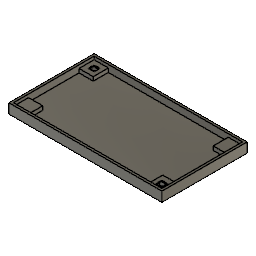
PCB_PDP_TD01_GP09 v1 (Autodesk Fusion 360 archive; units mm, degrees)
design "dessous"
Autodesk Fusion 360 part; units mm, degrees
sketch "Sketch1" plane through (0, 0, 0) normal (0, 0, 1) x (1, 0, 0)
  line L0 (-39.5, 22) -> (39.5, 22)
  line L1 (39.5, 22) -> (39.5, -22)
  line L2 (39.5, -22) -> (-39.5, -22)
  line L3 (-39.5, -22) -> (-39.5, 22)
  dimension "d1" = 79
  dimension "d2" = 44
  dimension "d3" = 39.5
  dimension "d4" = 22
  constraint horizontal L0
  constraint vertical L1
  constraint horizontal L2
  constraint vertical L3
  measures "d1" distance of L0.start L0.end
  measures "d2" distance of L0.start L2.end
  measures "d3" distance of origin L3
  measures "d4" distance of origin L0
extrude "Extrude1" add sketch "Sketch1" along normal blind 4.8
sketch "Sketch2" plane through (0, 0, 4.8) normal (0, 0, 1) x (-1, 0, 0)
  line L0 (39.5, 22) -> (-39.5, 22)
  line L1 (-39.5, 22) -> (-39.5, -22)
  line L2 (-39.5, -22) -> (39.5, -22)
  line L3 (39.5, -22) -> (39.5, 22)
  line L4 (38.3, -20.8) -> (-38.3, -20.8)
  line L5 (-38.3, -20.8) -> (-38.3, 20.8)
  line L6 (-38.3, 20.8) -> (38.3, 20.8)
  line L7 (38.3, 20.8) -> (38.3, -20.8)
  dimension "d7" = 76.6
  dimension "d8" = 41.6
  dimension "d9" = 1.2
  dimension "d10" = 1.2
  constraint horizontal L4
  constraint vertical L5
  constraint horizontal L6
  constraint vertical L7
  measures "d7" distance of L4.start L4.end
  measures "d8" distance of L4.start L6.end
  measures "d9" distance of L2 L4
  measures "d10" distance of L3 L7
extrude "Extrude2" cut sketch "Sketch2" against normal blind 3.6 contours L4 L5 L6 L7
sketch "Sketch3" plane through (0, 0, 1.2) normal (0, 0, 1) x (-1, 0, 0)
  line L0 (38.3, 20.8) -> (-38.3, 20.8)
  line L1 (-38.3, 20.8) -> (-38.3, -20.8)
  line L2 (-38.3, -20.8) -> (38.3, -20.8)
  line L3 (38.3, -20.8) -> (38.3, 20.8)
  circle A0 centre (-32.9, -15.4) radius 3.25
  line L4 (39.5, -22) -> (-39.5, -22)
  line L5 (-39.5, -22) -> (-39.5, 22)
  line L6 (39.5, 22) -> (39.5, -22)
  line L7 (-39.5, 22) -> (39.5, 22)
  circle A1 centre (32.9, 15.4) radius 3.25
  line L8 (39.5, 22) -> (39.5, -22)
  line L9 (-39.5, 22) -> (39.5, 22)
  dimension "d13" = 6.5
  dimension "d14" = 6.6
  dimension "d15" = 6.6
  dimension "d29" = 6.5
  dimension "d30" = 6.6
  dimension "d31" = 6.6
  measures "d13" diameter of A0
  measures "d14" distance of A0.centre L4
  measures "d15" distance of A0.centre L5
  measures "d29" diameter of A1
  measures "d30" distance of A1.centre L8
  measures "d31" distance of A1.centre L9
sketch "Sketch5" plane through (0, 0, 1.2) normal (0, 0, 1) x (1, 0, 0)
extrude "Extrude4" add sketch "Sketch3" along normal blind 2 contours A1
extrude "Extrude5" cut 1 faces at (-34.1709, -16.2087, 3.2) along direction (0, 0, -1) blind 2
sketch "Sketch6" plane through (0, 0, 0) normal (0, 0, -1) x (1, 0, 0)
  line L0 (39.5, 22) -> (-39.5, 22)
  line L1 (-39.5, 22) -> (-39.5, -22)
  line L2 (-39.5, -22) -> (39.5, -22)
  line L3 (39.5, -22) -> (39.5, 22)
  line L4 (-31.75, 15.4123) -> (-31.75, 18.5877)
  line L5 (-31.75, 18.5877) -> (-34.5, 20.1754)
  line L6 (-34.5, 20.1754) -> (-37.25, 18.5877)
  line L7 (-37.25, 18.5877) -> (-37.25, 15.4123)
  line L8 (-37.25, 15.4123) -> (-34.5, 13.8246)
  line L9 (-34.5, 13.8246) -> (-31.75, 15.4123)
  line L10 (-31.35, 22) -> (-31.35, 13.4246)
  line L11 (-31.35, 13.4246) -> (-39.5, 13.4246)
  point P0 (-34.5, 17)
  dimension "d36" = 2.75
  dimension "d37" = 5
  dimension "d38" = 5
  dimension "d50" = 0.4
  dimension "d51" = 0.4
  constraint parallel L1 L7
  constraint vertical L10
  constraint horizontal L11
  constraint coincident L1 L11.end
  constraint coincident L0 L10.start
  measures "d36" distance of P0 L9
  measures "d37" distance of L1 P0
  measures "d38" distance of L0 P0
  measures "d50" distance of L8.end L11
  measures "d51" distance of L4 L10
sketch "Sketch9" plane through (0, 0, 0) normal (0, 0, -1) x (1, 0, 0)
  line L0 (-37.25, -15.4123) -> (-37.25, -18.5877)
  line L1 (-37.25, -18.5877) -> (-34.5, -20.1754)
  line L2 (-34.5, -20.1754) -> (-31.75, -18.5877)
  line L3 (-31.75, -18.5877) -> (-31.75, -15.4123)
  line L4 (-31.75, -15.4123) -> (-34.5, -13.8246)
  line L5 (-34.5, -13.8246) -> (-37.25, -15.4123)
  line L6 (-39.5, 22) -> (-39.5, -22)
  line L7 (-39.5, -22) -> (39.5, -22)
  line L8 (-39.5, -13.0246) -> (-30.95, -13.0246)
  line L9 (-30.95, -13.0246) -> (-30.95, -22)
  point P0 (-34.5, -17)
  dimension "d61" = 2.75
  dimension "d62" = 5
  dimension "d63" = 5
  dimension "d64" = 0.8
  dimension "d65" = 0.8
  constraint parallel L3 L6
  constraint horizontal L8
  constraint vertical L9
  constraint coincident L7 L9.end
  constraint coincident L6 L8.start
  measures "d61" distance of P0 L5
  measures "d62" distance of P0 L6
  measures "d63" distance of P0 L7
  measures "d64" distance of L3 L9
  measures "d65" distance of L4.end L8
extrude "Extrude11" add sketch "Sketch9" against normal blind 3.2 contours L0 L1 L2 L3 L4 L5 | L6 L7 L8 L9
extrude "Extrude12" cut sketch "Sketch9" against normal blind 2.4 contours L0 L1 L2 L3 L4 L5
sketch "Sketch10" plane through (0, 0, 3.2) normal (0, 0, 1) x (-1, 0, 0)
  line L0 (38.3, -20.8) -> (38.3, -13.0246)
  line L1 (38.3, -13.0246) -> (30.95, -13.0246)
  line L2 (30.95, -13.0246) -> (30.95, -20.8)
  line L3 (30.95, -20.8) -> (38.3, -20.8)
  circle A0 centre (34.5, -17) radius 1.6
  line L4 (39.5, 22) -> (39.5, -22)
  line L5 (39.5, -22) -> (-39.5, -22)
  dimension "d70" = 3.2
  dimension "d71" = 5
  dimension "d72" = 5
  measures "d70" diameter of A0
  measures "d71" distance of A0.centre L4
  measures "d72" distance of A0.centre L5
extrude "Extrude13" cut sketch "Sketch10" against normal blind 3.2 contours A0
sketch "Sketch11" plane through (0, 0, 0) normal (0, 0, -1) x (1, 0, 0)
  line L0 (37.25, 15.4123) -> (37.25, 18.5877)
  line L1 (37.25, 18.5877) -> (34.5, 20.1754)
  line L2 (34.5, 20.1754) -> (31.75, 18.5877)
  line L3 (31.75, 18.5877) -> (31.75, 15.4123)
  line L4 (31.75, 15.4123) -> (34.5, 13.8246)
  line L5 (34.5, 13.8246) -> (37.25, 15.4123)
  line L6 (39.5, -22) -> (39.5, 22)
  line L7 (39.5, 22) -> (-39.5, 22)
  line L8 (39.5, 13.0246) -> (30.95, 13.0246)
  line L9 (30.95, 13.0246) -> (30.95, 22)
  point P0 (34.5, 17)
  dimension "d75" = 2.75
  dimension "d76" = 5
  dimension "d77" = 5
  dimension "d78" = 0.8
  dimension "d79" = 0.8
  constraint parallel L0 L6
  constraint horizontal L8
  constraint vertical L9
  constraint coincident L7 L9.end
  constraint coincident L6 L8.start
  measures "d75" distance of P0 L5
  measures "d76" distance of P0 L6
  measures "d77" distance of P0 L7
  measures "d78" distance of L4.end L8
  measures "d79" distance of L3 L9
extrude "Extrude14" add sketch "Sketch11" against normal blind 3.2 contours L0 L1 L2 L3 L4 L5 | L6 L7 L8 L9
extrude "Extrude15" cut sketch "Sketch11" against normal blind 2.4 contours L0 L1 L2 L3 L4 L5
sketch "Sketch12" plane through (0, 0, 3.2) normal (0, 0, 1) x (-1, 0, 0)
  line L0 (-38.3, 20.8) -> (-38.3, 13.0246)
  line L1 (-38.3, 13.0246) -> (-30.95, 13.0246)
  line L2 (-30.95, 13.0246) -> (-30.95, 20.8)
  line L3 (-30.95, 20.8) -> (-38.3, 20.8)
  circle A0 centre (-34.5, 17) radius 1.6
  line L4 (-39.5, -22) -> (-39.5, 22)
  line L5 (-39.5, 22) -> (39.5, 22)
  dimension "d84" = 3.2
  dimension "d85" = 5
  dimension "d86" = 5
  measures "d84" diameter of A0
  measures "d85" distance of A0.centre L4
  measures "d86" distance of A0.centre L5
extrude "Extrude16" cut sketch "Sketch12" against normal blind 3.2 contours A0
sketch "Sketch14" plane through (0, 0, 2.4) normal (0, 0, -1) x (1, 0, 0)
  circle A0 centre (-34.5, -17) radius 1.6
  line L0 (-34.5, -13.8246) -> (-37.25, -15.4123)
  line L1 (-37.25, -15.4123) -> (-37.25, -18.5877)
  line L2 (-37.25, -18.5877) -> (-34.5, -20.1754)
  line L3 (-34.5, -20.1754) -> (-31.75, -18.5877)
  line L4 (-31.75, -18.5877) -> (-31.75, -15.4123)
  line L5 (-31.75, -15.4123) -> (-34.5, -13.8246)
  line L6 (-37.25, -15.4123) -> (-31.75, -15.4123)
  line L7 (-31.75, -18.5877) -> (-37.25, -18.5877)
  line L8 (-36.1, -15.4123) -> (-36.1, -18.5877)
  line L9 (-32.9, -18.5877) -> (-32.9, -15.4123)
  constraint coincident L0.end L1.start
  constraint coincident L4.end L5.start
  constraint coincident L3.end L4.start
  constraint coincident L1.end L2.start
  constraint coincident L6 L8.start
  constraint coincident L7 L8.end
  constraint perpendicular L7 L8
  constraint coincident L7 L9.start
  constraint coincident L6 L9.end
  constraint perpendicular L6 L9
  constraint tangent A0 L9
  constraint tangent A0 L8
sketch "Sketch15" plane through (0, 0, 2.4) normal (0, 0, -1) x (1, 0, 0)
  circle A0 centre (34.5, 17) radius 1.6
  line L0 (34.5, 13.8246) -> (37.25, 15.4123)
  line L1 (37.25, 15.4123) -> (37.25, 18.5877)
  line L2 (37.25, 18.5877) -> (34.5, 20.1754)
  line L3 (34.5, 20.1754) -> (31.75, 18.5877)
  line L4 (31.75, 18.5877) -> (31.75, 15.4123)
  line L5 (31.75, 15.4123) -> (34.5, 13.8246)
  line L6 (31.75, 18.5877) -> (37.25, 18.5877)
  line L7 (37.25, 15.4123) -> (31.75, 15.4123)
  line L8 (32.9, 15.4123) -> (32.9, 18.5877)
  line L9 (36.1, 15.4123) -> (36.1, 18.5877)
  constraint coincident L3.end L4.start
  constraint coincident L1.end L2.start
  constraint coincident L0.end L1.start
  constraint coincident L4.end L5.start
  constraint coincident L7 L8.start
  constraint coincident L6 L8.end
  constraint perpendicular L6 L8
  constraint coincident L7 L9.start
  constraint coincident L6 L9.end
  constraint perpendicular L6 L9
  constraint tangent A0 L8
  constraint tangent A0 L9
extrude "Extrude17" cut sketch "Sketch14" sketch "Sketch15" against normal blind 0.5 contours A0 L7 L9 | A0 L6 L9 | A0 L6 L8 | A0 L7 L8 of sketch 2 contours A0 L7 L9 | A0 L6 L9 | A0 L6 L8 | A0 L7 L8
extrude "Extrude18" cut sketch "Sketch14" sketch "Sketch15" against normal blind 0.2 contours L4 L6 L7 L9 | L1 L6 L7 L8 of sketch 2 contours L1 L6 L7 L9 | L4 L6 L7 L8
extrude "Extrude19" add 4 faces at (35.4826, -19.117, 2.4) (35.4826, -14.883, 2.4) (-33.5174, 14.883, 2.4) (-33.5174, 19.117, 2.4) along direction (0, 0, -1) blind 0.1
sketch "Sketch16" plane through (0, 0, 1.2) normal (0, 0, 1) x (-1, 0, 0)
  line L0 (-30.95, 13.0246) -> (-38.3, 13.0246)
  line L1 (-38.3, 13.0246) -> (-38.3, -20.8)
  line L2 (-38.3, -20.8) -> (30.95, -20.8)
  line L3 (30.95, -20.8) -> (30.95, -13.0246)
  line L4 (30.95, -13.0246) -> (38.3, -13.0246)
  line L5 (38.3, -13.0246) -> (38.3, 20.8)
  line L6 (38.3, 20.8) -> (-30.95, 20.8)
  line L7 (-30.95, 20.8) -> (-30.95, 13.0246)
  line L8 (-30.95, -20.8) -> (-38.3, -20.8)
  line L9 (-38.3, -20.8) -> (-38.3, -13.025)
  line L10 (-38.3, -13.025) -> (-30.95, -13.025)
  line L11 (-30.95, -13.025) -> (-30.95, -20.8)
  line L12 (38.3, 20.8) -> (38.3, 13.025)
  line L13 (38.3, 13.025) -> (30.95, 13.025)
  line L14 (30.95, 20.8) -> (38.3, 20.8)
  line L15 (30.95, 13.025) -> (30.95, 20.8)
  dimension "d95" = 7.35
  dimension "d96" = 7.775
  dimension "d97" = 7.35
  dimension "d98" = 7.775
  constraint horizontal L8
  constraint vertical L9
  constraint horizontal L10
  constraint vertical L11
  constraint horizontal L13
  constraint vertical L15
  constraint horizontal L14
  constraint vertical L12
  constraint coincident L1.end L2.start
  constraint coincident L5.end L6.start
  measures "d95" distance of L8.start L1.end
  measures "d96" distance of L8.start L10.end
  measures "d97" distance of L13.end L12.end
  measures "d98" distance of L5.end L12.end
extrude "Extrude20" add sketch "Sketch16" along normal blind 2 contours L1 L2 L8 L9 L10 L11 | L5 L6 L12 L13 L14 L15
extrude "Extrude21" add 1 faces at (-13.1667, -7.3333, 0) along direction (0, 0, -1) blind 0.3

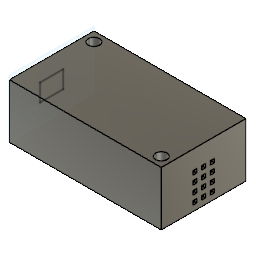
design "Couvercle"
Autodesk Fusion 360 part; units mm, degrees
sketch "Sketch1" plane through (0, 0, 0) normal (0, 0, 1) x (1, 0, 0)
  line L0 (-39.5, 22) -> (39.5, 22)
  line L1 (39.5, 22) -> (39.5, -22)
  line L2 (39.5, -22) -> (-39.5, -22)
  line L3 (-39.5, -22) -> (-39.5, 22)
  dimension "d1" = 79
  dimension "d2" = 44
  dimension "d3" = 39.5
  dimension "d4" = 22
  constraint horizontal L0
  constraint vertical L1
  constraint horizontal L2
  constraint vertical L3
  measures "d1" distance of L0.start L0.end
  measures "d2" distance of L0.start L2.end
  measures "d3" distance of origin L3
  measures "d4" distance of origin L0
extrude "Extrude1" add sketch "Sketch1" along normal blind 30.2
sketch "Sketch2" plane through (0, 0, 0) normal (0, 0, -1) x (1, 0, 0)
  line L0 (39.5, 22) -> (-39.5, 22)
  line L1 (-39.5, 22) -> (-39.5, -22)
  line L2 (-39.5, -22) -> (39.5, -22)
  line L3 (39.5, -22) -> (39.5, 22)
  line L4 (-38.3, 20.8) -> (38.3, 20.8)
  line L5 (38.3, 20.8) -> (38.3, -20.8)
  line L6 (38.3, -20.8) -> (-38.3, -20.8)
  line L7 (-38.3, -20.8) -> (-38.3, 20.8)
  dimension "d7" = 76.6
  dimension "d8" = 41.6
  dimension "d9" = 1.2
  dimension "d10" = 1.2
  constraint horizontal L4
  constraint vertical L5
  constraint horizontal L6
  constraint vertical L7
  measures "d7" distance of L4.start L4.end
  measures "d8" distance of L4.start L6.end
  measures "d9" distance of L1 L7
  measures "d10" distance of L0 L4
extrude "Extrude2" cut sketch "Sketch2" against normal blind 29 contours L4 L5 L6 L7
sketch "Sketch3" plane through (0, 0, 30.2) normal (0, 0, 1) x (-1, 0, 0)
  line L0 (39.5, 22) -> (-39.5, 22)
  line L1 (-39.5, 22) -> (-39.5, -22)
  line L2 (-39.5, -22) -> (39.5, -22)
  line L3 (39.5, -22) -> (39.5, 22)
  circle A0 centre (-34.5, 17) radius 4.15
  circle A1 centre (34.5, -17) radius 4.15
  line L4 (-34.5, 12.85) -> (-39.5, 12.85)
  line L5 (-30.35, 17) -> (-30.35, 22)
  line L6 (34.5, -12.85) -> (39.5, -12.85)
  line L7 (30.35, -17) -> (30.35, -22)
  circle A2 centre (-34.5, 17) radius 2.95
  circle A3 centre (34.5, -17) radius 2.95
  circle A4 centre (34.5, -17) radius 1.6
  circle A5 centre (-34.5, 17) radius 1.6
  circle A6 centre (31.5, 9) radius 3
  dimension "d13" = 8.3
  dimension "d14" = 5
  dimension "d15" = 5
  dimension "d16" = 8.3
  dimension "d17" = 5
  dimension "d18" = 5
  dimension "d23" = 5.9
  dimension "d24" = 5.9
  dimension "d29" = 3.2
  dimension "d30" = 3.2
  dimension "d35" = 6
  dimension "d36" = 8
  dimension "d37" = 13
  constraint coincident A0 L4.start
  constraint coincident L1 L4.end
  constraint tangent A0 L4
  constraint coincident A0 L5.start
  constraint coincident L0 L5.end
  constraint tangent A0 L5
  constraint parallel L0 L4
  constraint parallel L1 L5
  constraint coincident A1 L6.start
  constraint coincident L3 L6.end
  constraint tangent A1 L6
  constraint perpendicular L3 L6
  constraint coincident A1 L7.start
  constraint coincident L2 L7.end
  constraint tangent A1 L7
  constraint perpendicular L2 L7
  constraint concentric A0 A2
  constraint concentric A1 A3
  constraint concentric A3 A4
  constraint concentric A2 A5
  measures "d13" diameter of A0
  measures "d14" distance of L0 A0.centre
  measures "d15" distance of L1 A0.centre
  measures "d16" diameter of A1
  measures "d17" distance of L3 A1.centre
  measures "d18" distance of L2 A1.centre
  measures "d23" diameter of A2
  measures "d24" diameter of A3
  measures "d29" diameter of A4
  measures "d30" diameter of A5
  measures "d35" diameter of A6
  measures "d36" distance of L3 A6.centre
  measures "d37" distance of L0 A6.centre
extrude "Extrude3" add sketch "Sketch3" against normal blind 30.2 contours L2 L3 A1 L6 L7 | A1 | A3 | A4
extrude "Extrude4" add sketch "Sketch3" against normal blind 30.2 contours L0 L1 A0 L4 L5 | A0 | A2 | A5
extrude "Extrude5" cut sketch "Sketch3" against normal blind 24.2 contours A2 | A5
extrude "Extrude6" cut sketch "Sketch3" against normal blind 24.2 contours A3 | A4
extrude "Extrude7" cut sketch "Sketch3" against normal blind 30.2 contours A4
extrude "Extrude8" cut sketch "Sketch3" against normal blind 30.2 contours A5
sketch "Sketch4" plane through (39.5, 0, 0) normal (1, 0, 0) x (0, 1, 0)
  line L0 (-22, 0) -> (22, 0)
  line L1 (22, 0) -> (22, 30.2)
  line L2 (22, 30.2) -> (-22, 30.2)
  line L3 (-22, 30.2) -> (-22, 0)
  line L4 (-5.5, 18.5) -> (-3.5, 18.5)
  line L5 (-3.5, 18.5) -> (-3.5, 16.5)
  line L6 (-3.5, 16.5) -> (-5.5, 16.5)
  line L7 (-5.5, 16.5) -> (-5.5, 18.5)
  line L8 (3.5, 18.5) -> (5.5, 18.5)
  line L9 (5.5, 18.5) -> (5.5, 16.5)
  line L10 (5.5, 16.5) -> (3.5, 16.5)
  line L11 (3.5, 16.5) -> (3.5, 18.5)
  line L12 (-1, 18.5) -> (1, 18.5)
  line L13 (1, 18.5) -> (1, 16.5)
  line L14 (1, 16.5) -> (-1, 16.5)
  line L15 (-1, 16.5) -> (-1, 18.5)
  line L16 (-5.5, 14) -> (-3.5, 14)
  line L17 (-3.5, 14) -> (-3.5, 12)
  line L18 (-3.5, 12) -> (-5.5, 12)
  line L19 (-5.5, 12) -> (-5.5, 14)
  line L20 (-1, 14) -> (1, 14)
  line L21 (1, 14) -> (1, 12)
  line L22 (1, 12) -> (-1, 12)
  line L23 (-1, 12) -> (-1, 14)
  line L24 (3.5, 14) -> (5.5, 14)
  line L25 (5.5, 14) -> (5.5, 12)
  line L26 (5.5, 12) -> (3.5, 12)
  line L27 (3.5, 12) -> (3.5, 14)
  line L28 (-5.5, 9.5) -> (-3.5, 9.5)
  line L29 (-3.5, 9.5) -> (-3.5, 7.5)
  line L30 (-3.5, 7.5) -> (-5.5, 7.5)
  line L31 (-5.5, 7.5) -> (-5.5, 9.5)
  line L32 (-1, 9.5) -> (1, 9.5)
  line L33 (1, 9.5) -> (1, 7.5)
  line L34 (1, 7.5) -> (-1, 7.5)
  line L35 (-1, 7.5) -> (-1, 9.5)
  line L36 (3.5, 9.5) -> (5.5, 9.5)
  line L37 (5.5, 9.5) -> (5.5, 7.5)
  line L38 (5.5, 7.5) -> (3.5, 7.5)
  line L39 (3.5, 7.5) -> (3.5, 9.5)
  line L40 (-5.5, 5) -> (-3.5, 5)
  line L41 (-3.5, 5) -> (-3.5, 3)
  line L42 (-3.5, 3) -> (-5.5, 3)
  line L43 (-5.5, 3) -> (-5.5, 5)
  line L44 (-1, 5) -> (1, 5)
  line L45 (1, 5) -> (1, 3)
  line L46 (1, 3) -> (-1, 3)
  line L47 (-1, 3) -> (-1, 5)
  line L48 (3.5, 5) -> (5.5, 5)
  line L49 (5.5, 5) -> (5.5, 3)
  line L50 (5.5, 3) -> (3.5, 3)
  line L51 (3.5, 3) -> (3.5, 5)
  dimension "d40" = 2
  dimension "d41" = 2
  dimension "d61" = 16.5
  dimension "d62" = 2
  dimension "d63" = 2
  dimension "d64" = 16.5
  dimension "d66" = 2
  dimension "d67" = 2
  dimension "d69" = 2.5
  dimension "d70" = 16.5
  dimension "d71" = 2.5
  dimension "d72" = 2.5
  dimension "d73" = 2.5
  dimension "d74" = 2
  dimension "d75" = 2
  dimension "d76" = 2.5
  dimension "d77" = 2.5
  dimension "d78" = 16.5
  dimension "d79" = 2.5
  dimension "d80" = 2.5
  dimension "d81" = 2.5
  dimension "d82" = 2
  dimension "d83" = 2
  dimension "d84" = 2.5
  dimension "d85" = 16.5
  dimension "d86" = 16.5
  dimension "d87" = 16.5
  dimension "d88" = 2.5
  dimension "d89" = 2.5
  dimension "d90" = 2.5
  dimension "d91" = 2.5
  dimension "d92" = 16.5
  dimension "d93" = 2.5
  dimension "d94" = 3
  dimension "d95" = 3
  dimension "d96" = 3
  dimension "d97" = 5
  dimension "d98" = 5
  dimension "d99" = 18.5
  dimension "d100" = 18.5
  dimension "d101" = 9.5
  dimension "d102" = 12
  dimension "d103" = 25.5
  dimension "d104" = 25.5
  dimension "d105" = 7.5
  dimension "d106" = 23
  dimension "d107" = 25.5
  dimension "d108" = 21
  constraint horizontal L4
  constraint vertical L5
  constraint horizontal L6
  constraint vertical L7
  constraint horizontal L8
  constraint vertical L9
  constraint horizontal L10
  constraint vertical L11
  constraint horizontal L12
  constraint vertical L13
  constraint horizontal L14
  constraint vertical L15
  constraint horizontal L16
  constraint vertical L17
  constraint horizontal L18
  constraint vertical L19
  constraint horizontal L20
  constraint vertical L21
  constraint horizontal L22
  constraint vertical L23
  constraint horizontal L24
  constraint vertical L25
  constraint horizontal L26
  constraint vertical L27
  constraint horizontal L28
  constraint vertical L29
  constraint horizontal L30
  constraint vertical L31
  constraint horizontal L32
  constraint vertical L33
  constraint horizontal L34
  constraint vertical L35
  constraint horizontal L36
  constraint vertical L37
  constraint horizontal L38
  constraint vertical L39
  constraint horizontal L40
  constraint vertical L41
  constraint horizontal L42
  constraint vertical L43
  constraint horizontal L44
  constraint vertical L45
  constraint horizontal L46
  constraint vertical L47
  constraint horizontal L48
  constraint vertical L49
  constraint horizontal L50
  constraint vertical L51
  measures "d40" distance of L4.start L4.end
  measures "d41" distance of L4.start L6.end
  measures "d61" distance of L3 L7
  measures "d62" distance of L8.start L8.end
  measures "d63" distance of L8.end L9.end
  measures "d64" distance of L1 L9
  measures "d66" distance of L12.start L12.end
  measures "d67" distance of L12.end L13.end
  measures "d69" distance of L11 L13
  measures "d70" distance of L3 L16.start
  measures "d71" distance of L6 L16
  measures "d72" distance of L14 L20
  measures "d73" distance of L17 L23
  measures "d74" distance of L24.start L24.end
  measures "d75" distance of L24.start L26.end
  measures "d76" distance of L21 L27
  measures "d77" distance of L10 L24
  measures "d78" distance of L3 L31
  measures "d79" distance of L18 L28
  measures "d80" distance of L22 L32
  measures "d81" distance of L29 L35
  measures "d82" distance of L36.start L36.end
  measures "d83" distance of L36 L38
  measures "d84" distance of L26.end L36
  measures "d85" distance of L1 L37
  measures "d86" distance of L1 L25
  measures "d87" distance of L3 L43
  measures "d88" distance of L30.end L40
  measures "d89" distance of L34 L44
  measures "d90" distance of L41 L47
  measures "d91" distance of L45 L51
  measures "d92" distance of L1 L49
  measures "d93" distance of L38 L48
  measures "d94" distance of L0 L42
  measures "d95" distance of L0 L46
  measures "d96" distance of L0 L50
  measures "d97" distance of L0 L48
  measures "d98" distance of L0 L44
  measures "d99" distance of L0 L4
  measures "d100" distance of L0 L12
  measures "d101" distance of L0 L32
  measures "d102" distance of L0 L18
  measures "d103" distance of L1 L17
  measures "d104" distance of L1 L29
  measures "d105" distance of L0 L30
  measures "d106" distance of L3 L33
  measures "d107" distance of L1 L41
  measures "d108" distance of L1 L45
extrude "Extrude10" cut sketch "Sketch4" against normal blind 1.2 contours L4 L5 L6 L7 | L8 L9 L10 L11 | L12 L13 L14 L15 | L16 L17 L18 L19 | L20 L21 L22 L23 | L24 L25 L26 L27 | L28 L29 L30 L31 | L32 L33 L34 L35 | L36 L37 L38 L39 | L40 L41 L42 L43 | L44 L45 L46 L47 | L48 L49 L50 L51
sketch "Sketch5" plane through (-39.5, 0, 0) normal (-1, 0, 0) x (0, -1, 0)
  line L0 (-22, 0) -> (22, 0)
  line L1 (22, 0) -> (22, 30.2)
  line L2 (22, 30.2) -> (-22, 30.2)
  line L3 (-22, 30.2) -> (-22, 0)
  circle A0 centre (9.6787, 7.232) radius 2.25
  line L4 (11.8, 6.1713) -> (9.6787, 4.05)
  line L5 (9.6787, 4.05) -> (7.5574, 6.1713)
  line L6 (9.6787, 4.05) -> (9.6787, 7.232)
  dimension "d111" = 4.5
  dimension "d112" = 3
  dimension "d113" = 3
  dimension "d131" = 10.2
  dimension "d132" = 4.05
  constraint perpendicular L4 L5
  constraint tangent A0 L4
  constraint tangent A0 L5
  constraint coincident A0.centre L6.end
  constraint parallel L1 L6
  measures "d111" diameter of A0
  measures "d112" distance of L4.start L4.end
  measures "d113" distance of L4.end L5.end
  measures "d131" distance of L1 L4.start
  measures "d132" distance of L0 L4.end
extrude "Extrude11" cut sketch "Sketch5" against normal blind 1.2 contours A0 | A0 L5 L6 | A0 L4 L6
sketch "Sketch6" plane through (-39.5, 0, 0) normal (-1, 0, 0) x (0, -1, 0)
  line L0 (9.6787, 4.05) -> (8.0877, 5.641)
  arc A0 (11.2697, 5.641) -> (8.0877, 5.641) centre (9.6787, 7.232) ccw
  line L1 (11.2697, 5.641) -> (9.6787, 4.05)
  line L2 (-22, 0) -> (22, 0)
  line L3 (22, 0) -> (22, 30.2)
  line L4 (22, 30.2) -> (-22, 30.2)
  line L5 (-22, 30.2) -> (-22, 0)
  line L6 (-6, 18.9) -> (6, 18.9)
  line L7 (6, 18.9) -> (6, 9.9)
  line L8 (6, 9.9) -> (-6, 9.9)
  line L9 (-6, 9.9) -> (-6, 18.9)
  dimension "d121" = 9
  dimension "d122" = 16
  dimension "d123" = 16
  dimension "d168" = 9.9
  constraint horizontal L6
  constraint vertical L7
  constraint horizontal L8
  constraint vertical L9
  measures "d121" distance of L6 L8
  measures "d122" distance of L3 L7
  measures "d123" distance of L5 L9
  measures "d168" distance of L2 L8
extrude "Extrude12" cut sketch "Sketch6" against normal blind 1.2 contours L6 L7 L8 L9
sketch "Sketch11" plane through (0, 0, 6) normal (0, 0, 1) x (-1, 0, 0)
  circle A0 centre (-34.5, 17) radius 1.6
  circle A1 centre (-34.5, 17) radius 2.95
  line L0 (-32.9, 19.4784) -> (-32.9, 14.5216)
  line L1 (-36.1, 19.4784) -> (-36.1, 14.5216)
  line L2 (-39.5, -22) -> (-39.5, 22)
  line L3 (-36.1, 18.6) -> (-32.9, 18.6)
  line L4 (-36.1, 15.4) -> (-32.9, 15.4)
  constraint coincident A1 L0.start
  constraint coincident A1 L0.end
  constraint coincident A1 L1.start
  constraint coincident A1 L1.end
  constraint tangent A0 L1
  constraint tangent A0 L0
  constraint parallel L1 L2
  constraint parallel L0 L2
  constraint coincident L1 L3.start
  constraint coincident L0 L3.end
  constraint perpendicular L0 L3
  constraint coincident L1 L4.start
  constraint coincident L0 L4.end
  constraint perpendicular L0 L4
  constraint tangent A0 L3
  constraint tangent A0 L4
sketch "Sketch10" plane through (0, 22, 0) normal (0, 1, 0) x (-1, 0, 0)
  line L0 (39.5, 30.2) -> (-39.5, 30.2)
  line L1 (-39.5, 30.2) -> (-39.5, 0)
  line L2 (-39.5, 0) -> (39.5, 0)
  line L3 (39.5, 0) -> (39.5, 30.2)
  line L4 (-33, 13) -> (33, 13) construction
  line L5 (33, 13) -> (33, 22.2) construction
  line L6 (33, 22.2) -> (-33, 22.2) construction
  line L7 (-33, 22.2) -> (-33, 13) construction
  dimension "d147" = 8
  dimension "d148" = 6.5
  dimension "d149" = 6.5
  dimension "d150" = 8
  dimension "d151" = 13
  text T0 "TD01 GP09" font "Arial" height 8 align centre middle in box 66 x 9.2 at (-33, 13) x (1, 0) y (0, 1) spacing 1 kerned
  constraint parallel L0 L6
  measures "d148" distance of L1 L7
  measures "d149" distance of L3 L5
  measures "d150" distance of L0 L6
  measures "d151" distance of L2 L4
extrude "Extrude13" add sketch "Sketch10" along normal blind 0.4 text T0
extrude "Extrude14" cut sketch "Sketch11" against normal blind 0.6 contours A0 L0 L4 | A0 L0 L3 | A0 L1 L3 | A0 L1 L4
extrude "Extrude15" cut sketch "Sketch11" against normal blind 0.3 contours A1 L0 L1 L3
extrude "Extrude16" cut sketch "Sketch11" against normal blind 0.3 contours A1 L0 L1 L4
sketch "Sketch12" plane through (0, 0, 30.2) normal (0, 0, 1) x (-1, 0, 0)
  circle A0 centre (34.5, -17) radius 2.95
  circle A1 centre (-34.5, 17) radius 2.95
  line L0 (39.5, 22) -> (-39.5, 22)
  line L1 (-39.5, 22) -> (-39.5, -22)
  line L2 (-39.5, -22) -> (39.5, -22)
  line L3 (39.5, -22) -> (39.5, 22)
  line L4 (39.5, -22) -> (-39.5, -22)
  line L5 (-39.5, -22) -> (-39.5, 22)
  line L6 (-39.5, 22) -> (39.5, 22)
  line L7 (39.5, 22) -> (39.5, -22)
  constraint horizontal L4
  constraint vertical L5
  constraint horizontal L6
  constraint vertical L7
  constraint coincident L0.end L1.start
  constraint coincident L2.end L3.start
extrude "Extrude17" cut sketch "Sketch12" against normal blind 3.2
sketch "Sketch13" plane through (0, 0, 27) normal (0, 0, 1) x (-1, 0, 0)
  line L0 (30.35, -17) -> (30.35, -20.8)
  line L1 (30.35, -20.8) -> (-38.3, -20.8)
  line L2 (-38.3, -20.8) -> (-38.3, 12.85)
  line L3 (-38.3, 12.85) -> (-34.5, 12.85)
  arc A0 (-34.5, 12.85) -> (-30.35, 17) centre (-34.5, 17) ccw
  line L4 (-30.35, 17) -> (-30.35, 20.8)
  line L5 (-30.35, 20.8) -> (38.3, 20.8)
  line L6 (38.3, 20.8) -> (38.3, -12.85)
  line L7 (38.3, -12.85) -> (34.5, -12.85)
  arc A1 (34.5, -12.85) -> (30.35, -17) centre (34.5, -17) ccw
  circle A2 centre (-34.5, 17) radius 2.95
  circle A3 centre (34.5, -17) radius 2.95
  line L8 (39.5, 22) -> (-39.5, 22)
  line L9 (-39.5, 22) -> (-39.5, -22)
  line L10 (-39.5, -22) -> (39.5, -22)
  line L11 (39.5, -22) -> (39.5, 22)
  line L12 (39.5, -22) -> (-39.5, -22)
  line L13 (-39.5, -22) -> (-39.5, 22)
  line L14 (-39.5, 22) -> (39.5, 22)
  line L15 (39.5, 22) -> (39.5, -22)
  constraint horizontal L12
  constraint vertical L13
  constraint horizontal L14
  constraint vertical L15
  constraint coincident L8.end L9.start
  constraint coincident L10.end L11.start
extrude "Extrude18" add sketch "Sketch13" along normal blind 1.2 contours L0 L1 L2 L3 A0 L4 L5 L6 L7 A1 | L8 L9 L10 L11 L12 L13 L14 L15
sketch "Sketch14" plane through (0, 0, 6) normal (0, 0, 1) x (-1, 0, 0)
  circle A0 centre (34.5, -17) radius 1.6
  circle A1 centre (34.5, -17) radius 2.95
  line L0 (36.1, -19.4784) -> (36.1, -14.5216)
  line L1 (32.9, -14.5216) -> (32.9, -19.4784)
  line L2 (32.9, -18.6) -> (36.1, -18.6)
  line L3 (32.9, -15.4) -> (36.1, -15.4)
  line L4 (39.5, -22) -> (39.5, 22)
  line L5 (-39.5, -22) -> (39.5, -22)
  constraint coincident A1 L0.start
  constraint coincident A1 L0.end
  constraint coincident A1 L1.start
  constraint coincident A1 L1.end
  constraint parallel L0 L1
  constraint coincident L1 L2.start
  constraint coincident L0 L2.end
  constraint horizontal L2
  constraint coincident L1 L3.start
  constraint parallel L1 L4
  constraint parallel L3 L5
  constraint tangent A0 L1
  constraint tangent A0 L2
  constraint tangent A0 L3
  constraint tangent A0 L0
  constraint coincident L0 L3.end
extrude "Extrude19" cut sketch "Sketch14" against normal blind 0.6 contours A0 L0 L2 | A0 L0 L3 | A0 L1 L3 | A0 L1 L2
extrude "Extrude20" cut sketch "Sketch14" against normal blind 0.3 contours A1 L0 L1 L3 | A1 L0 L1 L2
